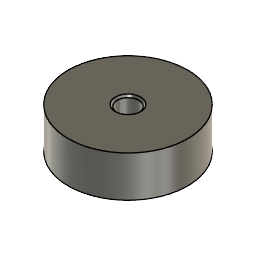
card-dispenser (Autodesk Fusion 360 archive; units mm, degrees)
design "card-dispenser-wheels"
part number: 2026-07-26-23-07-40-715
Autodesk Fusion 360 part; units mm, degrees
sketch "Sketch1" plane through (0, 0, 0) normal (0, 0, 1) x (1, 0, 0)
  circle A0 centre (0, 0) radius 16
  circle A1 centre (0, 0) radius 2.9
  dimension "d1" = 32
  dimension "d2" = 5.8
  constraint coincident A0.centre A1.centre
  measures "d1" diameter of A0
  measures "d2" diameter of A1
extrude "Extrude1" add sketch "Sketch1" along normal blind 11
chamfer "Chamfer1" distance 0.5 angle 45 2 edges at (-2.7037, 1.0487, 11) (-2.7037, 1.0487, 0) tangent chain off
